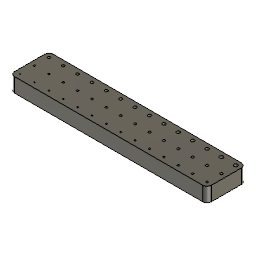
PL Hypodermic Needle Hole Sizer (Autodesk Fusion 360 design; units mm, degrees)
Autodesk Fusion 360 part; units mm, degrees
sketch "Sketch1" plane through (0, 0, 0) normal (0, 0, 1) x (1, 0, 0)
  circle A0 centre (0, 0) radius 0.74
  circle A1 centre (10, 0) radius 0.765
  circle A2 centre (20, 0) radius 0.79
  circle A3 centre (30, 0) radius 0.815
  circle A4 centre (40, 0) radius 0.84
  line L0 (0, 0) -> (10, 0) construction
  line L1 (10, 0) -> (20, 0) construction
  line L2 (20, 0) -> (30, 0) construction
  line L3 (30, 0) -> (40, 0) construction
  circle A5 centre (50, 0) radius 0.865
  circle A6 centre (60, 0) radius 0.89
  circle A7 centre (70, 0) radius 0.915
  line L4 (40, 0) -> (50, 0) construction
  line L5 (50, 0) -> (60, 0) construction
  line L6 (60, 0) -> (70, 0) construction
  line L7 (-50, 0) -> (-40, 0) construction
  line L8 (-40, 0) -> (-30, 0) construction
  circle A8 centre (-40, 0) radius 0.64
  line L9 (-10, 0) -> (0, 0) construction
  circle A9 centre (-50, 0) radius 0.615
  circle A10 centre (-30, 0) radius 0.665
  circle A11 centre (-60, 0) radius 0.59
  circle A12 centre (-20, 0) radius 0.69
  line L10 (-30, 0) -> (-20, 0) construction
  line L11 (-60, 0) -> (-50, 0) construction
  line L12 (-20, 0) -> (-10, 0) construction
  circle A13 centre (-10, 0) radius 0.715
  line L13 (0, 0) -> (0, 10) construction
  circle A14 centre (-40, 10) radius 0.95
  line L14 (-50, 10) -> (-40, 10) construction
  line L15 (20, 10) -> (30, 10) construction
  circle A15 centre (20, 10) radius 1.1
  line L16 (-30, 10) -> (-20, 10) construction
  circle A16 centre (0, 10) radius 1.05
  circle A17 centre (-50, 10) radius 0.925
  line L17 (-60, 10) -> (-50, 10) construction
  line L18 (40, 10) -> (50, 10) construction
  line L19 (-40, 10) -> (-30, 10) construction
  circle A18 centre (10, 10) radius 1.075
  circle A19 centre (-30, 10) radius 0.975
  line L20 (-20, 10) -> (-10, 10) construction
  circle A20 centre (60, 10) radius 1.2
  circle A21 centre (70, 10) radius 1.225
  line L21 (60, 10) -> (70, 10) construction
  circle A22 centre (30, 10) radius 1.125
  line L22 (50, 10) -> (60, 10) construction
  circle A23 centre (40, 10) radius 1.15
  circle A24 centre (50, 10) radius 1.175
  line L23 (30, 10) -> (40, 10) construction
  circle A25 centre (-10, 10) radius 1.025
  line L24 (-10, 10) -> (0, 10) construction
  line L25 (0, 10) -> (10, 10) construction
  circle A26 centre (-20, 10) radius 1
  circle A27 centre (-60, 10) radius 0.9
  line L26 (10, 10) -> (20, 10) construction
  line L27 (0, 0) -> (0, -10) construction
  line L28 (0, -10) -> (10, -10) construction
  circle A28 centre (30, -10) radius 0.6
  circle A29 centre (20, -10) radius 0.575
  circle A30 centre (40, -10) radius 0.625
  line L29 (50, -10) -> (60, -10) construction
  circle A31 centre (70, -10) radius 0.7
  circle A32 centre (10, -10) radius 0.55
  line L30 (20, -10) -> (30, -10) construction
  circle A33 centre (0, -10) radius 0.525
  line L31 (-20, -10) -> (-10, -10) construction
  circle A34 centre (-10, -10) radius 0.5
  circle A35 centre (-20, -10) radius 0.475
  line L32 (-10, -10) -> (0, -10) construction
  circle A36 centre (-40, -10) radius 0.425
  circle A37 centre (-60, -10) radius 0.375
  line L33 (-60, -10) -> (-50, -10) construction
  line L34 (-30, -10) -> (-20, -10) construction
  circle A38 centre (-50, -10) radius 0.4
  line L35 (-40, -10) -> (-30, -10) construction
  line L36 (-50, -10) -> (-40, -10) construction
  circle A39 centre (-30, -10) radius 0.45
  circle A40 centre (50, -10) radius 0.65
  line L37 (10, -10) -> (20, -10) construction
  line L38 (40, -10) -> (50, -10) construction
  line L39 (60, -10) -> (70, -10) construction
  line L40 (30, -10) -> (40, -10) construction
  circle A41 centre (60, -10) radius 0.675
  line L41 (73.5, 13.5) -> (-63.5, 13.5)
  line L42 (-63.5, 13.5) -> (-63.5, -13.5)
  line L43 (-63.5, -13.5) -> (73.5, -13.5)
  line L44 (73.5, -13.5) -> (73.5, 13.5)
  line L45 (73.5, 13.5) -> (-63.5, -13.5) construction
  line L46 (-63.5, 13.5) -> (73.5, -13.5) construction
  point P0 (-60, 0)
  point P1 (-60, 10)
  point P2 (0, 10)
  point P3 (0, 10)
  point P4 (0, -10)
  point P5 (-60, -10)
  point P6 (0, -10)
  point P7 (0, -10)
  point P8 (5, 0)
  dimension "d1" = 1.48
  dimension "d2" = 10
  dimension "d3" = 1.53
  dimension "d4" = 1.58
  dimension "d5" = 1.63
  dimension "d6" = 1.68
  dimension "d7" = 1.73
  dimension "d8" = 1.78
  dimension "d9" = 1.83
  dimension "d10" = 1.18
  dimension "d11" = 10
  dimension "d12" = 1.23
  dimension "d13" = 1.28
  dimension "d14" = 1.33
  dimension "d15" = 1.38
  dimension "d16" = 1.43
  dimension "d18" = 10
  dimension "d19" = 2.1
  dimension "d20" = 10
  dimension "d21" = 2.15
  dimension "d22" = 2.2
  dimension "d23" = 2.25
  dimension "d24" = 2.3
  dimension "d25" = 2.35
  dimension "d26" = 2.4
  dimension "d27" = 2.45
  dimension "d28" = 1.8
  dimension "d29" = 10
  dimension "d30" = 1.85
  dimension "d31" = 1.9
  dimension "d32" = 1.95
  dimension "d33" = 2
  dimension "d34" = 2.05
  dimension "d35" = 1.05
  dimension "d36" = 10
  dimension "d37" = 1.1
  dimension "d38" = 1.15
  dimension "d39" = 1.2
  dimension "d40" = 1.25
  dimension "d41" = 1.3
  dimension "d42" = 1.35
  dimension "d43" = 1.4
  dimension "d44" = 0.75
  dimension "d45" = 10
  dimension "d46" = 0.8
  dimension "d47" = 0.85
  dimension "d48" = 0.9
  dimension "d49" = 0.95
  dimension "d50" = 1
  dimension "d51" = 137
  dimension "d52" = 27
  constraint coincident A0.centre L0.start
  constraint coincident A1.centre L0.end
  constraint horizontal L0
  constraint coincident A2.centre L1.end
  constraint coincident A3.centre L2.end
  constraint coincident A4.centre L3.end
  constraint horizontal L3
  constraint horizontal L2
  constraint horizontal L1
  constraint equal L0 L1
  constraint equal L1 L2
  constraint equal L2 L3
  constraint coincident A5.centre L4.end
  constraint coincident A6.centre L5.end
  constraint horizontal L5
  constraint coincident A7.centre L6.end
  constraint parallel L5 L6
  constraint horizontal L4
  constraint equal L3 L4
  constraint equal L3 L5
  constraint equal L5 L6
  constraint coincident P0 A11.centre
  constraint coincident L7.start A9.centre
  constraint horizontal L11
  constraint coincident L7.end L8.start
  constraint coincident L8.end A10.centre
  constraint coincident A12.centre L10.end
  constraint horizontal L10
  constraint horizontal L8
  constraint horizontal L7
  constraint equal L7 L11
  constraint equal L7 L8
  constraint equal L8 L10
  constraint coincident L9.start L12.end
  constraint horizontal L9
  constraint horizontal L12
  constraint equal L10 L12
  constraint equal L9 L10
  constraint perpendicular L0 L13
  constraint coincident P3 P2
  constraint coincident A18.centre L25.end
  constraint horizontal L25
  constraint coincident L15.start A15.centre
  constraint coincident L15.end A22.centre
  constraint coincident L18.start A23.centre
  constraint horizontal L23
  constraint horizontal L15
  constraint horizontal L26
  constraint equal L25 L26
  constraint equal L15 L26
  constraint equal L15 L23
  constraint coincident L18.end L22.start
  constraint coincident A20.centre L21.start
  constraint horizontal L22
  constraint coincident A21.centre L21.end
  constraint parallel L21 L22
  constraint horizontal L18
  constraint equal L18 L23
  constraint equal L22 L23
  constraint equal L21 L22
  constraint coincident P1 L17.start
  constraint coincident L14.start A17.centre
  constraint horizontal L17
  constraint coincident A14.centre L14.end
  constraint coincident L16.start L19.end
  constraint coincident L16.end L20.start
  constraint horizontal L16
  constraint horizontal L19
  constraint horizontal L14
  constraint equal L14 L17
  constraint equal L14 L19
  constraint equal L16 L19
  constraint coincident L20.end A25.centre
  constraint horizontal L24
  constraint horizontal L20
  constraint equal L16 L20
  constraint equal L16 L24
  constraint perpendicular L9 L27
  constraint equal L13 L27
  constraint coincident P7 P6
  constraint coincident L28.end A32.centre
  constraint horizontal L28
  constraint coincident A29.centre L30.start
  constraint coincident A28.centre L30.end
  constraint coincident A30.centre L38.start
  constraint horizontal L40
  constraint horizontal L30
  constraint horizontal L37
  constraint equal L28 L37
  constraint equal L30 L37
  constraint equal L30 L40
  constraint coincident L29.start A40.centre
  constraint coincident L29.end L39.start
  constraint horizontal L29
  constraint coincident A31.centre L39.end
  constraint parallel L29 L39
  constraint horizontal L38
  constraint equal L38 L40
  constraint equal L29 L40
  constraint equal L29 L39
  constraint coincident P5 A37.centre
  constraint coincident L33.end A38.centre
  constraint horizontal L33
  constraint coincident A36.centre L35.start
  constraint coincident L34.start L35.end
  constraint coincident L31.start A35.centre
  constraint horizontal L34
  constraint horizontal L35
  constraint horizontal L36
  constraint equal L33 L36
  constraint equal L35 L36
  constraint equal L34 L35
  constraint coincident L31.end A34.centre
  constraint horizontal L32
  constraint horizontal L31
  constraint equal L31 L34
  constraint equal L32 L34
  constraint horizontal L41
  constraint perpendicular L41 L42
  constraint parallel L41 L43
  constraint parallel L42 L44
  constraint coincident L45 P8
  constraint coincident L46 P8
  constraint midpoint L0 P8
  measures "d1" diameter of A0
  measures "d2" distance of A0.centre A1.centre
  measures "d3" diameter of A1
  measures "d4" diameter of A2
  measures "d5" diameter of A3
  measures "d6" diameter of A4
  measures "d7" diameter of A5
  measures "d8" diameter of A6
  measures "d9" diameter of A7
  measures "d10" diameter of A11
  measures "d11" distance of P0 L7.start
  measures "d12" diameter of A9
  measures "d13" diameter of A8
  measures "d14" diameter of A10
  measures "d15" diameter of A12
  measures "d16" diameter of A13
  measures "d18" distance of A0.centre P3
  measures "d19" diameter of A16
  measures "d20" distance of P3 A18.centre
  measures "d21" diameter of A18
  measures "d22" diameter of A15
  measures "d23" diameter of A22
  measures "d24" diameter of A23
  measures "d25" diameter of A24
  measures "d26" diameter of A20
  measures "d27" diameter of A21
  measures "d28" diameter of A27
  measures "d29" distance of P1 L14.start
  measures "d30" diameter of A17
  measures "d31" diameter of A14
  measures "d32" diameter of A19
  measures "d33" diameter of A26
  measures "d34" diameter of A25
  measures "d35" diameter of A33
  measures "d36" distance of P7 L28.end
  measures "d37" diameter of A32
  measures "d38" diameter of A29
  measures "d39" diameter of A28
  measures "d40" diameter of A30
  measures "d41" diameter of A40
  measures "d42" diameter of A41
  measures "d43" diameter of A31
  measures "d44" diameter of A37
  measures "d45" distance of P5 L33.end
  measures "d46" diameter of A38
  measures "d47" diameter of A36
  measures "d48" diameter of A39
  measures "d49" diameter of A35
  measures "d50" diameter of A34
  measures "d51" distance of L42.end L43.end
  measures "d52" distance of L41.end L42.end
extrude "Extrude1" add sketch "Sketch1" along normal blind 10
fillet "Fillet1" radius 3 4 edges at (73.5, -13.5, 5) (73.5, 13.5, 5) (-63.5, -13.5, 5) (-63.5, 13.5, 5)
equation "d2 = d18"
equation "d3 = d1 + 0.05 mm"
equation "d4 = d3 + 0.05 mm"
equation "d5 = d4 + 0.05 mm"
equation "d6 = d5 + 0.05 mm"
equation "d7 = d6 + 0.05 mm"
equation "d8 = d7 + 0.05 mm"
equation "d9 = d8 + 0.05 mm"
equation "d10 = d12 - 0.05 mm"
equation "d11 = d2"
equation "d12 = d13 - 0.05 mm"
equation "d13 = d14 - 0.05 mm"
equation "d14 = d15 - 0.05 mm"
equation "d15 = d16 - 0.05 mm"
equation "d16 = d1 - 0.05 mm"
equation "d20 = d2"
equation "d21 = d19 + 0.05 mm"
equation "d22 = d19 + 0.1 mm"
equation "d23 = d19 + 0.15 mm"
equation "d24 = d19 + 0.2 mm"
equation "d25 = d19 + 0.25 mm"
equation "d26 = d19 + 0.3 mm"
equation "d27 = d19 + 0.35 mm"
equation "d28 = d19 - 0.3 mm"
equation "d29 = d2"
equation "d30 = d19 - 0.25 mm"
equation "d31 = d19 - 0.2 mm"
equation "d32 = d19 - 0.15 mm"
equation "d33 = d19 - 0.1 mm"
equation "d34 = d19 - 0.05 mm"
equation "d36 = d2"
equation "d37 = d35 + 0.05 mm"
equation "d38 = d37 + 0.05 mm"
equation "d39 = d38 + 0.05 mm"
equation "d40 = d39 + 0.05 mm"
equation "d41 = d40 + 0.05 mm"
equation "d42 = d41 + 0.05 mm"
equation "d43 = d42 + 0.05 mm"
equation "d44 = d46 - 0.05 mm"
equation "d45 = d2"
equation "d46 = d47 - 0.05 mm"
equation "d47 = d48 - 0.05 mm"
equation "d48 = d49 - 0.05 mm"
equation "d49 = d50 - 0.05 mm"
equation "d50 = d35 - 0.05 mm"
